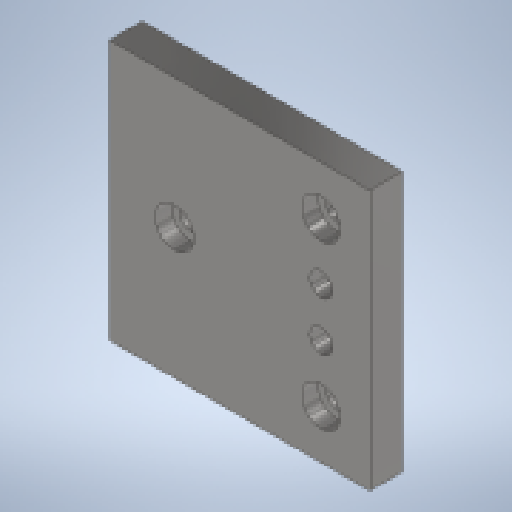
# Autodesk Inventor part: HCMUTE-CDT23-DE_GA_LOADCELL
Saved by Autodesk Inventor 2023 (Build 270158000, 158)
## iProperties
Created: 2023-10-14
Part Number: HCMUTE-CDT23-DE_GA_LOADCELL
Material: Stainless Steel
Document SubType Name: Modeling
Designer: havie
Density: 8 g/cm^3
Appearance: Steel - Polished
Author: havie
Autodesk Inventor part; units mm, degrees
ref_plane "YZ Plane" through (0, 0, 0) normal (1, 0, 0) x (0, 1, 0)
ref_plane "XZ Plane" through (0, 0, 0) normal (0, 1, 0) x (-1, 0, 0)
ref_plane "XY Plane" through (0, 0, 0) normal (0, 0, 1) x (1, 0, 0)
sketch "Sketch1" plane through (0, 0, 0) normal (0, 0, 1) x (1, 0, 0)
  line L0 (40, -40) -> (-40, -40)
  line L1 (-40, -40) -> (-40, 40)
  line L2 (-40, 40) -> (40, 40)
  line L3 (40, 40) -> (40, -40)
  line L4 (40, -40) -> (-40, 40) construction
  line L5 (-40, -40) -> (40, 40) construction
  point P0 (0, 0)
  dimension "d1" = 80
  dimension "d2" = 80
  constraints: 12 end point, 2 midpoint, 2 parallel, 1 horizontal, 1 perpendicular
  measures "d1" distance of L0.start L0.end
  measures "d2" distance of L0.end L1.end
extrude "Extrusion1" add sketch "Sketch1" along normal mid plane 10
sketch "Sketch2" plane through (0, 0, 5) normal (0, 0, 1) x (1, 0, 0)
  line L0 (-40, 40) -> (-40, -40) projected
  line L1 (40, 40) -> (-40, 40) projected
  line L2 (40, -40) -> (40, 40) projected
  point P0 (0, 0)
  point P1 (25, 25)
  point P2 (25, -25)
  point P3 (-20, 0)
  point P4 (-40, 0)
  dimension "d27" = 15
  dimension "d31" = 15
  dimension "d32" = 50
  dimension "d33" = 40
  dimension "d34" = 20
  constraints: 1 midpoint, 1 vertical alignment
  measures "d27" distance from line of L2 point (25, 25)
  measures "d31" distance from line of L1 point (25, 25)
  measures "d32" distance of point (25, -25) point (25, 25)
  measures "d33" distance from line of L1 point (-20, 0)
  measures "d34" distance of point (-40, 0) point (-20, 0)
hole "Hole1" at (25, 25, 5) at (25, -25, 5) at (-20, 0, 5) direction (0, 0, -1) diameter 7 depth 17.1 tip angle 118 counterbore diameter 12 counterbore depth 5
sketch "Sketch3" plane through (0, 0, -5) normal (0, 0, -1) x (-1, 0, 0)
  line L0 (-40, -40) -> (40, -40) projected
  line L1 (56, 0) -> (-56, 0) construction
  circle A0 centre (-25, 25) radius 3.5 projected
  point P0 (0, 0)
  point P1 (-25, -7.5)
  point P2 (-25, 7.5)
  dimension "d28" = 0
  dimension "d29" = 15
  dimension "d30" = 7.5
  constraints: 1 vertical alignment
  measures "d28" horizontal distance of point (-25, -7.5) A0.centre
  measures "d29" distance of point (-25, 7.5) point (-25, -7.5)
  measures "d30" vertical distance of point (0, 0) point (-25, -7.5)
hole "Hole2" at (25, -7.5, -5) at (25, 7.5, -5) direction (0, 0, 1) diameter 7 depth 17.1 tip angle 118
body "Solid1"
